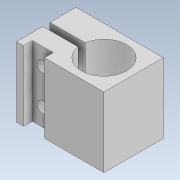
# Autodesk Inventor part: ACCROCHE SUR ACIER
Saved by Autodesk Inventor 2020 (Build 240168000, 168)
## iProperties
Created: 2020-07-01
Part Number: ACCROCHE SUR ACIER
Material: Generic
Document SubType Name: Modeling
Designer: Admin
Density: 1 g/cm^3
Appearance: Default
Author: Admin
Autodesk Inventor part; units mm, degrees
ref_plane "YZ Plane" through (0, 0, 0) normal (1, 0, 0) x (0, 1, 0)
ref_plane "XZ Plane" through (0, 0, 0) normal (0, 1, 0) x (-1, 0, 0)
ref_plane "XY Plane" through (0, 0, 0) normal (0, 0, 1) x (1, 0, 0)
sketch "Sketch1" plane through (0, 0, 0) normal (0, 1, 0) x (-1, 0, 0)
  line L0 (0, 0) -> (25, 0)
  line L1 (25, 0) -> (25, -17)
  line L2 (25, -17) -> (0, -17)
  line L3 (0, -17) -> (0, 0)
  dimension "d0" = 17
  dimension "d1" = 25
  constraints: 8 end point, 2 parallel, 1 horizontal, 1 perpendicular
  measures "d0" distance of L2.end L0.start
  measures "d1" distance of L1.end L2.end
extrude "Extrusion1" add sketch "Sketch1" along normal blind 20
sketch "Sketch2" plane through (0, 20, 0) normal (0, 1, 0) x (1, 0, 0)
  circle A0 centre (-8.5, 8.5) radius 5
  line L0 (-25, 0) -> (0, 0) projected
  line L1 (0, 0) -> (0, 17) projected
  dimension "d4" = 10
  dimension "d5" = 8.5
  dimension "d6" = 8.5
  constraints: 1 centre point
  measures "d4" diameter of A0
  measures "d5" distance from line of L0 A0.centre
  measures "d6" distance from line of L1 A0.centre
extrude "Extrusion2" cut sketch "Sketch2" against normal through all
sketch "Sketch3" plane through (0, 20, 0) normal (0, 1, 0) x (1, 0, 0)
  circle A0 centre (-8.5, 8.5) radius 6.5
  line L0 (-25, 0) -> (0, 0) projected
  line L1 (0, 0) -> (0, 17) projected
  dimension "d9" = 13
  dimension "d10" = 8.5
  dimension "d11" = 8.5
  constraints: 1 centre point
  measures "d9" diameter of A0
  measures "d10" distance from line of L0 A0.centre
  measures "d11" distance from line of L1 A0.centre
extrude "Extrusion3" cut sketch "Sketch3" against normal blind 10
sketch "Sketch4" plane through (0, 20, 0) normal (0, 1, 0) x (1, 0, 0)
  line L0 (-25, 17) -> (-25, 0) projected
  line L1 (-25, 7.5) -> (-12, 7.5)
  line L2 (-12, 7.5) -> (-12, 9.5)
  line L3 (-12, 9.5) -> (-25, 9.5)
  line L4 (-25, 9.5) -> (-25, 7.5)
  line L5 (-25, 0) -> (0, 0) projected
  dimension "d14" = 2
  dimension "d15" = 7.5
  dimension "d16" = 13
  constraints: 8 end point, 2 parallel, 1 horizontal, 1 perpendicular, 1 point on line
  measures "d14" distance of L1.end L2.end
  measures "d15" distance between parallel lines of L5 L1
  measures "d16" distance of L1.start L1.end
extrude "Extrusion4" cut sketch "Sketch4" against normal through all
sketch "Sketch5" plane through (0, 20, 0) normal (0, 1, 0) x (1, 0, 0)
  line L0 (-23, 0) -> (-17, 0)
  line L1 (-17, 0) -> (-17, 2.5)
  line L2 (-17, 2.5) -> (-23, 2.5)
  line L3 (-23, 2.5) -> (-23, 0)
  line L4 (-25, 7.5) -> (-25, 0) projected
  line L5 (-25, 0) -> (0, 0) projected
  dimension "d19" = 6
  dimension "d20" = 2.5
  dimension "d21" = 2
  constraints: 8 end point, 2 parallel, 1 horizontal, 1 perpendicular, 1 point on line
  measures "d19" distance of L1.end L2.end
  measures "d20" distance of L2.end L0.start
  measures "d21" distance between parallel lines of L4 L3
extrude "Extrusion5" cut sketch "Sketch5" against normal through all
sketch "Sketch6" plane through (0, 0, -17) normal (0, 0, -1) x (-1, 0, 0)
  circle A0 centre (20, 15) radius 1.6
  circle A1 centre (20, 5) radius 1.6
  line L0 (25, 0) -> (25, 20) projected
  line L1 (0, 20) -> (25, 20) projected
  line L2 (0, 0) -> (25, 0) projected
  dimension "d24" = 3.2
  dimension "d25" = 3.2
  dimension "d26" = 5
  dimension "d27" = 5
  dimension "d28" = 5
  dimension "d29" = 5
  constraints: 2 centre point
  measures "d24" diameter of A0
  measures "d25" diameter of A1
  measures "d26" distance from line of L0 A0.centre
  measures "d27" distance from line of L0 A1.centre
  measures "d28" distance from line of L1 A0.centre
  measures "d29" distance from line of L2 A1.centre
extrude "Extrusion6" cut sketch "Sketch6" against normal through all
sketch "Sketch7" plane through (0, 0, -17) normal (0, 0, -1) x (-1, 0, 0)
  circle A0 centre (20, 5) radius 2.9
  circle A1 centre (20, 15) radius 2.9
  line L0 (25, 0) -> (25, 20) projected
  line L1 (0, 0) -> (25, 0) projected
  line L2 (0, 20) -> (25, 20) projected
  dimension "d32" = 5.8
  dimension "d33" = 5.8
  dimension "d34" = 5
  dimension "d35" = 5
  dimension "d36" = 5
  dimension "d37" = 5
  constraints: 2 centre point
  measures "d32" diameter of A0
  measures "d33" diameter of A1
  measures "d34" distance from line of L0 A0.centre
  measures "d35" distance from line of L0 A1.centre
  measures "d36" distance from line of L1 A0.centre
  measures "d37" distance from line of L2 A1.centre
extrude "Extrusion7" cut sketch "Sketch7" against normal blind 3
body "Solid1"
